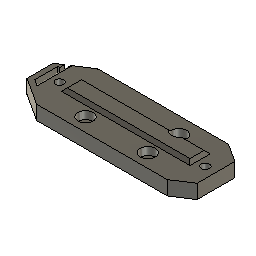
sfs_mount (Autodesk Fusion 360 design; units mm, degrees)
Autodesk Fusion 360 part; units mm, degrees
note: some values were not read from the file. Set by a fixed rule: which sketch regions a step uses.
sketch "Sketch1" plane through (0, 0, 0) normal (0, 0, 1) x (1, 0, 0)
  line L0 (0, 0) -> (51.8, 0)
  line L1 (51.8, 0) -> (51.8, 24.3)
  line L2 (51.8, 24.3) -> (0, 24.3)
  line L3 (0, 24.3) -> (0, 0)
  circle A0 centre (14, 5.4) radius 1.6
  circle A1 centre (38.7, 17.8) radius 1.6
  circle A2 centre (38.7, 5.4) radius 1.6
  line L4 (38.7, 17.8) -> (38.7, 5.4) construction
  line L5 (38.7, 5.4) -> (14, 5.4) construction
  line L6 (25.9, 24.3) -> (25.9, 0) construction
  circle A3 centre (38.7, 17.8) radius 3
  circle A4 centre (38.7, 5.4) radius 3
  circle A5 centre (14, 5.4) radius 3
  line L7 (51.8, 0) -> (59, 4.65)
  line L8 (59, 4.65) -> (59, 19.65)
  line L9 (59, 19.65) -> (51.8, 24.3)
  line L10 (0, 0) -> (-7.2, 4.65)
  line L11 (-7.2, 4.65) -> (-7.2, 19.65)
  line L12 (-7.2, 19.65) -> (0, 24.3)
  circle A6 centre (54.8, 12.15) radius 1.6
  circle A7 centre (-3, 12.15) radius 1.6
  line L13 (0, 12.15) -> (51.8, 12.15) construction
  circle A8 centre (-3, 12.15) radius 3
  circle A9 centre (54.8, 12.15) radius 3
  line L14 (-7.2, 4.65) -> (-10.8, 6.975)
  line L15 (-10.8, 6.975) -> (-10.8, 17.325)
  line L16 (-10.8, 17.325) -> (-8, 19.1333)
  line L17 (-8, 19.1333) -> (-8, 17.1333)
  line L18 (-8, 17.1333) -> (-8.8, 17.1333)
  line L19 (-8.8, 17.1333) -> (-8.8, 8.0642)
  line L20 (-8.8, 8.0642) -> (-7.2, 7.0308)
  dimension "d1" = 3.2
  dimension "d2" = 24.7
  dimension "d3" = 12.4
  dimension "d4" = 51.8
  dimension "d5" = 24.3
  dimension "d6" = 11.9
  dimension "d7" = 5.4
  dimension "d8" = 6
  dimension "d13" = 3.2
  dimension "d14" = 1.2
  dimension "d15" = 1.2
  dimension "d16" = 15
  dimension "d35" = 2
  dimension "d36" = 2
  dimension "d37" = 1.6
  dimension "d38" = 0.8
  dimension "d39" = 2
  constraint horizontal L0
  constraint vertical L1
  constraint horizontal L2
  constraint vertical L3
  constraint coincident L0.start L3.end
  constraint equal A0 A1
  constraint equal A0 A2
  constraint coincident A1.centre L4.start
  constraint vertical L4
  constraint coincident A2.centre L4.end
  constraint perpendicular L4 L5
  constraint coincident A0.centre L5.end
  constraint midpoint L2 L6.start
  constraint midpoint L0 L6.end
  constraint concentric A1 A3
  constraint concentric A2 A4
  constraint concentric A0 A5
  constraint equal A3 A4
  constraint equal A4 A5
  constraint perpendicular L0 L8
  constraint perpendicular L0 L11
  constraint midpoint L3 L13.start
  constraint midpoint L1 L13.end
  constraint coincident A6.centre L13
  constraint coincident A7.centre L13
  constraint equal A6 A7
  constraint concentric A7 A8
  constraint concentric A6 A9
  constraint equal A4 A9
  constraint equal A8 A9
  constraint tangent L3 A8
  constraint tangent L1 A9
  constraint equal L7 L9
  constraint equal L10 L12
  constraint equal L8 L11
  constraint parallel L10 L14
  constraint parallel L11 L15
  constraint parallel L15 L17
  constraint perpendicular L17 L18
  constraint perpendicular L18 L19
  constraint coincident L11 L20.end
  constraint parallel L14 L20
  constraint collinear L12 L16
  measures "d1" diameter of A0
  measures "d2" distance of A0.centre L4
  measures "d3" distance of A1.centre A2.centre
  measures "d4" distance of L1 L3
  measures "d5" distance of L0.end L1.end
  measures "d6" distance of A0.centre L6
  measures "d7" distance of L0 L5
  measures "d8" diameter of A3
  measures "d13" diameter of A6
  measures "d14" distance of L11 A8
  measures "d15" distance of L8 A9
  measures "d16" distance of L7.end L8.end
  measures "d35" distance of L14 L20
  measures "d36" distance of L15 L19
  measures "d37" distance of L11 L19
  measures "d38" distance of L17.end L18.end
  measures "d39" distance of L16.end L17.end
extrude "Extrude1" add sketch "Sketch1" along normal blind 5.6 contours L0 L1 L2 L3 | L3 L10 L11 L12 | L1 L7 L8 L9 | L11 L14 L15 L16 L17 L18 L19 L20
extrude "Extrude2" add sketch "Sketch1" along normal blind 2.5 contours A3 | A4 | A5
extrude "Extrude3" add sketch "Sketch1" along normal blind 2.6 from surface at 3 contours A8 | A9
sketch "Sketch2" plane through (0, 0, 5.6) normal (0, 0, 1) x (-1, 0, 0)
  circle A0 centre (-14, -5.4) radius 3
  circle A1 centre (-38.7, -17.8) radius 3
  circle A2 centre (-38.7, -5.4) radius 3
  line L0 (0, 0) -> (-51.8, 0)
  line L1 (-51.8, -24.3) -> (0, -24.3)
  line L2 (0, -24.3) -> (7.2, -19.65)
  line L3 (7.2, -19.65) -> (7.2, -7.0308)
  line L4 (10.8, -6.975) -> (0, 0)
  line L5 (-59.2, -13.3404) -> (7.2, -13.3404) construction
  line L6 (-59.2, -17.3404) -> (7.2, -17.3404)
  line L7 (7.2, -9.3404) -> (-59.2, -9.3404)
  line L8 (-51.5, -9.3404) -> (-51.5, -17.3404)
  line L9 (-0.5, -9.3404) -> (-0.5, -17.3404)
  line L10 (7.2, -7.0308) -> (8.8, -8.0642)
  line L11 (8.8, -8.0642) -> (8.8, -17.1333)
  line L12 (8.8, -17.1333) -> (8, -17.1333)
  line L13 (8, -17.1333) -> (8, -19.1333)
  line L14 (8, -19.1333) -> (10.8, -17.325)
  line L15 (10.8, -17.325) -> (10.8, -6.975)
  line L16 (-51.8, 0) -> (-59, -4.65)
  line L17 (-59, -4.65) -> (-59, -19.65)
  line L18 (-59, -19.65) -> (-51.8, -24.3)
  circle A3 centre (-54.8, -12.15) radius 1.6
  circle A4 centre (3, -12.15) radius 1.6
  dimension "d20" = 8
  constraint midpoint L3 L5.end
  constraint coincident L3 L6.end
  constraint perpendicular L3 L6
  constraint coincident L3 L7.start
  constraint symmetric L5 L6 L7
  constraint coincident L7 L8.start
  constraint coincident L6 L8.end
  constraint perpendicular L6 L8
  constraint coincident L7 L9.start
  constraint coincident L6 L9.end
  constraint perpendicular L6 L9
  measures "d20" distance of L6 L7
extrude "Extrude4" add sketch "Sketch2" along normal blind 1.2 contours A1 L6 L7 L8 L9
chamfer "Chamfer1" distance 1.2 angle 45 5 edges at (18.1177, 17.3404, 6.8) (26, 9.3404, 6.8) (46.5823, 17.3404, 6.8) (51.5, 13.3404, 6.8) (0.5, 13.3404, 6.8)
fillet "Fillet1" radius 1 2 edges at (-8.8, 12.5988, 0) (-7.2, 13.3404, 5.6)
equation "d7 = 4.2 mm + 1.2 mm"
equation "d15 = d14"
equation "d36 = d35"
equation "d39 = d35"
